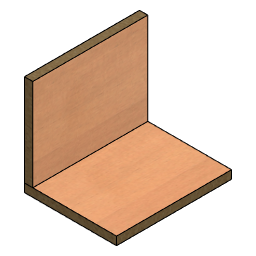
Test Assembly (Autodesk Fusion 360 design; units mm, degrees)
Autodesk Fusion 360 part; units mm, degrees
sketch "Sketch1" plane through (0, 0, 0) normal (0, 1, 0) x (1, 0, 0)
  line L0 (0, 0) -> (200, 0)
  line L1 (200, 0) -> (200, -18)
  line L2 (200, -18) -> (0, -18)
  line L3 (0, -18) -> (0, 0)
  line L4 (0, -218) -> (18, -218)
  line L5 (18, -218) -> (18, -18)
  line L6 (18, -18) -> (0, -18)
  line L7 (0, -18) -> (0, -218)
  dimension "d1" = 200
  dimension "d2" = 18
  dimension "d3" = 18
  dimension "d4" = 200
  constraint horizontal L0
  constraint vertical L1
  constraint horizontal L2
  constraint vertical L3
  constraint coincident L0.start L3.end
  constraint horizontal L4
  constraint vertical L5
  constraint horizontal L6
  constraint vertical L7
  constraint coincident L2.end L3.start
  measures "d1" distance of L0.start L0.end
  measures "d2" distance of L0.start L2.end
  measures "d3" distance of L4.start L4.end
  measures "d4" distance of L4.start L2.end
extrude "Extrude1" add sketch "Sketch1" along normal blind 250 contours L0 L1 L2 L3 L6 makes body 1
extrude "Extrude2" add sketch "Sketch1" along normal blind 250 separate body contours L2 L4 L5 L6 L7 makes body 2
copy_body "Body->Comp1" bodies 1 removing the originals makes body 3 in component "Body1"
copy_body "Body->Comp2" bodies 2 removing the originals makes body 4 in component "Body2"
component "Body1" placed x (1, 0, 0) y (0, 1, 0) z (0, 0, 1) at (0, 0, 0)
component "Body2" placed x (1, 0, 0) y (0, 1, 0) z (0, 0, 1) at (0, 0, 0)
equation "Length = 250 mm"
equation "d6 = Length"
equation "d8 = Length"
